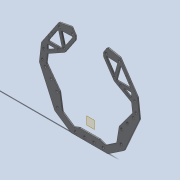
# Autodesk Inventor part: HeadMount2
Saved by Autodesk Inventor 2020 (Build 240168000, 168)
## iProperties
Created: 2021-07-03
Part Number: HeadMount2
Material: Generic
Document SubType Name: Sheet Metal
Designer: Val
Density: 1 g/cm^3
Sheet Metal Rule: Default
Appearance: Default
Author: Val
Autodesk Inventor part; units mm, degrees
ref_plane "YZ Plane" through (0, 0, 0) normal (1, 0, 0) x (0, 1, 0)
ref_plane "XZ Plane" through (0, 0, 0) normal (0, 1, 0) x (-1, 0, 0)
ref_plane "XY Plane" through (0, 0, 0) normal (0, 0, 1) x (1, 0, 0)
ref_plane "HeadMountPlane" through (0, 0, 3.048) normal (0, 0, 1) x (1, 0, 0)
sketch "Base" plane through (0, 0, 3.048) normal (0, 0, 1) x (1, 0, 0)
  line L0 (-84.8386, 199.7574) -> (-34.2356, 209.5937)
  line L1 (-34.2356, 209.5937) -> (-30.7591, 191.7089)
  line L2 (-30.7591, 191.7089) -> (-68.2682, 136.0994)
  line L3 (-68.2682, 136.0994) -> (-116.7076, 108.9972)
  line L4 (-116.7076, 108.9972) -> (-119.5296, 84.4705)
  line L5 (-119.5296, 84.4705) -> (-82.4198, 34.2032)
  line L6 (-82.4198, 34.2032) -> (-75.2404, -10.1332)
  line L7 (-44.3373, -30.9776) -> (-75.2404, -10.1332)
  line L8 (-138.9788, 78.2294) -> (-96.4615, -17.266)
  line L9 (-96.4615, -17.266) -> (-51.1674, -47.8172)
  line L10 (-44.3373, -30.9776) -> (-27.7964, -24.9572)
  line L11 (-27.7964, -24.9572) -> (0, -24.9572)
  line L12 (-51.1674, -47.8172) -> (0, -47.8172)
  line L13 (-133.255, 127.9772) -> (-138.9788, 78.2294)
  line L14 (0, -99.2994) -> (0, 261.0758) construction
  line L15 (-194.5703, 0) -> (194.5703, 0) construction
  line L16 (-84.8386, 199.7574) -> (-133.255, 127.9772)
  line L17 (84.8386, 199.7574) -> (34.2356, 209.5937)
  line L18 (34.2356, 209.5937) -> (30.7591, 191.7089)
  line L19 (30.7591, 191.7089) -> (68.2682, 136.0994)
  line L20 (68.2682, 136.0994) -> (116.7076, 108.9972)
  line L21 (116.7076, 108.9972) -> (119.5296, 84.4705)
  line L22 (119.5296, 84.4705) -> (82.4198, 34.2032)
  line L23 (82.4198, 34.2032) -> (75.2404, -10.1332)
  line L24 (44.3373, -30.9776) -> (75.2404, -10.1332)
  line L25 (138.9788, 78.2294) -> (96.4615, -17.266)
  line L26 (96.4615, -17.266) -> (51.1674, -47.8172)
  line L27 (44.3373, -30.9776) -> (27.7964, -24.9572)
  line L28 (27.7964, -24.9572) -> (0, -24.9572)
  line L29 (51.1674, -47.8172) -> (0, -47.8172)
  line L30 (133.255, 127.9772) -> (138.9788, 78.2294)
  line L31 (84.8386, 199.7574) -> (133.255, 127.9772)
  dimension "d61" = 160
  dimension "d63" = 126
  dimension "d65" = 17.78
  dimension "d66" = 22.86
  dimension "d67" = 137
  dimension "d68" = 125.791
  dimension "d70" = 34
  dimension "d71" = 11
  dimension "d74" = 83.437
  dimension "d75" = 99.198
  dimension "d76" = 114
  dimension "d77" = 24.9572
  dimension "d78" = 18.6084
  dimension "d79" = 49.3346
  dimension "d80" = 46.2853
  dimension "d81" = 82.6042
  dimension "d82" = 57.1022
  dimension "d83" = 20.7312
  dimension "d84" = 110.5412
  dimension "d85" = 116.1758
  dimension "d86" = 40.5476
  dimension "d87" = 175.1495
  dimension "d88" = 80.4922
  dimension "d89" = 197.3813
  dimension "d90" = 0
  dimension "d91" = 0
  measures "d61" angle of L11 L10
  measures "d63" angle of L10 L7
  measures "d65" distance between parallel lines of L9 L7
  measures "d66" distance between parallel lines of L12 L11
  measures "d67" angle of L4 L5
  measures "d68" angle of L3 L4
  measures "d70" angle of L14 L2
  measures "d71" angle of L14 L1
  measures "d74" angle of L15 L30
  measures "d75" angle of L15 L6
  measures "d76" angle of L15 L8
  measures "d77" distance between parallel lines of L15 L11
  measures "d78" distance between parallel lines of L21 L30
  measures "d79" distance between parallel lines of L19 L31
  measures "d80" distance from line of L15.end L30
  measures "d81" distance from line of L15.end L25
  measures "d82" distance from line of L15.end L20
  measures "d83" distance from line of L15.end L31
  measures "d84" distance from line of L15.end L22
  measures "d85" distance from line of L15.end L23
  measures "d86" distance from line of L15.end L26
  measures "d87" distance from line of L15.end L17
  measures "d88" distance from line of L15.end L27
  measures "d89" distance from line of L15.end L18
  measures "d90" distance from line of L11.end L14
  measures "d91" distance from line of L12.end L14
extrude "Plate2" add sketch "Base" along normal blind 3.175
sketch "MountHoles" plane through (0, 0, 6.223) normal (0, 0, 1) x (1, 0, 0)
  circle A0 centre (82.6068, 190.1381) radius 2.7051 construction
  circle A1 centre (126.1495, 116.4039) radius 2.7051 construction
  circle A2 centre (-126.1493, 116.4039) radius 2.7051 construction
  circle A3 centre (-82.6065, 190.1381) radius 2.2682 construction
  circle A4 centre (-82.6065, 190.1381) radius 3.175
  circle A5 centre (-126.1493, 116.4039) radius 3.175
  circle A6 centre (82.6068, 190.1381) radius 3.175
  circle A7 centre (126.1495, 116.4039) radius 3.175
  point P0 (0, 0)
  dimension "d172" = 6.35
  dimension "d173" = 6.35
  dimension "d174" = 6.35
  dimension "d175" = 6.35
  constraints: 4 centre point, 4 coincident
  measures "d172" diameter of A4
  measures "d173" diameter of A5
  measures "d174" diameter of A6
  measures "d175" diameter of A7
extrude "MountHolesFeature" cut sketch "MountHoles" against normal blind 3.175
sketch "EndCut" plane through (0, 0, 6.223) normal (0, 0, 1) x (1, 0, 0)
  line L0 (-84.8386, 199.7574) -> (-34.2356, 209.5937) projected
  line L1 (-49.4756, 206.6313) -> (-35.3576, 184.8914)
  line L2 (-30.7591, 191.7089) -> (-68.2682, 136.0994) projected
  line L3 (-34.2356, 209.5937) -> (-30.7591, 191.7089) projected
  point P0 (0, 0)
  dimension "d94" = 22
  dimension "d95" = 15.24
  constraints: 2 end point, 2 point on line
  measures "d94" angle of L3 L1
  measures "d95" horizontal distance of L0.end L1.start
extrude "EndCutFeature" cut sketch "EndCut" against normal blind 3.175
mirror "EndCutMirrorFeature" about plane through (0, 0, 0) normal (1, 0, 0) of "EndCutFeature"
sketch "Pattern" plane through (0, 0, 6.223) normal (0, 0, 1) x (1, 0, 0)
  line L0 (-27.7964, -24.9572) -> (27.7964, -24.9572) construction
  line L1 (0, -24.9572) -> (0, -47.8172)
  line L2 (51.1674, -47.8172) -> (-51.1674, -47.8172) construction
  circle A0 centre (-38.1, -39.3974) radius 3.175
  circle A1 centre (-88.1853, -6.0444) radius 3.175
  circle A2 centre (-122.5543, 75.0981) radius 3.175
  line L3 (-115.1093, 140.5729) -> (-74.9005, 140.5729)
  line L4 (-74.9005, 140.5729) -> (-86.3732, 183.1759)
  line L5 (-86.3732, 183.1759) -> (-115.1093, 140.5729)
  line L6 (-68.9795, 149.3513) -> (-78.184, 183.5316)
  line L7 (-78.184, 183.5316) -> (-44.9508, 184.9752)
  line L8 (-44.9508, 184.9752) -> (-68.9795, 149.3513)
  line L9 (-90.9552, 132.5729) -> (-116.7076, 132.5729)
  line L10 (-116.7076, 132.5729) -> (-116.7076, 118.1643)
  line L11 (-116.7076, 118.1643) -> (-90.9552, 132.5729)
  line L12 (-68.2682, 136.0994) -> (-116.7076, 108.9972) projected
  circle A3 centre (-90.0071, 31.0111) radius 3.175
  circle A4 centre (-106.2807, 53.0546) radius 3.175
  circle A5 centre (-12.7, -39.3974) radius 3.175
  line L13 (-44.3373, -30.9776) -> (-51.1674, -47.8172) construction
  line L14 (-38.1, -39.3974) -> (-12.7, -39.3974) construction
  line L15 (-51.1674, -47.8172) -> (-96.4615, -17.266) construction
  line L16 (-75.2404, -10.1332) -> (-96.4615, -17.266) construction
  line L17 (-82.4198, 34.2032) -> (-75.2404, -10.1332) construction
  line L18 (-96.4615, -17.266) -> (-138.9788, 78.2294) construction
  line L19 (-122.5543, 75.0981) -> (-90.0071, 31.0111) construction
  line L20 (-119.5296, 84.4705) -> (-82.4198, 34.2032) construction
  line L21 (-116.7076, 108.9972) -> (-119.5296, 84.4705) projected
  line L22 (-119.5296, 84.4705) -> (-138.9788, 78.2294) construction
  line L23 (-35.3576, 184.8914) -> (-68.2682, 136.0994) projected
  line L24 (-35.3576, 184.8914) -> (-49.4756, 206.6313) projected
  line L25 (-116.7076, 118.1643) -> (-116.7076, 108.9972) construction
  line L26 (-133.255, 127.9772) -> (-84.8386, 199.7574) projected
  line L27 (-84.8386, 199.7574) -> (-49.4756, 206.6313) projected
  line L28 (-74.9005, 140.5729) -> (-68.2682, 136.0994) construction
  line L29 (-86.3732, 183.1759) -> (-78.184, 183.5316) construction
  circle A6 centre (-129.2811, 89.1837) radius 3.175
  line L30 (-126.1493, 116.4039) -> (-129.2811, 89.1837) construction
  circle A7 centre (-126.1493, 116.4039) radius 3.175 projected
  circle A8 centre (-82.6065, 190.1381) radius 2.2682 projected
  point P0 (0, 0)
  dimension "d121" = 8.4198
  dimension "d122" = 8.4198
  dimension "d123" = 25.4
  dimension "d124" = 12.7
  dimension "d125" = 12.1249
  dimension "d126" = 12.1249
  dimension "d127" = 8
  dimension "d128" = 8
  dimension "d129" = 8
  dimension "d130" = 8
  dimension "d134" = 8
  dimension "d135" = 8
  dimension "d136" = 8
  dimension "d137" = 8
  dimension "d139" = 8
  dimension "d141" = 8
  dimension "d143" = 8
  dimension "d161" = 27.3997
  dimension "d162" = 27.3997
  dimension "d176" = 6.35
  dimension "d178" = 2.487
  constraints: 38 end point, 8 parallel, 7 centre point, 6 equal radius, 3 midpoint, 2 horizontal, 2 perpendicular, 1 coincident, 1 collinear, 1 vertical
  measures "d121" distance between parallel lines of L2 L14
  measures "d122" distance from line of L13.start L14
  measures "d123" distance of L14.start L14.end
  measures "d124" distance from line of L1 L14.end
  measures "d125" distance from line of L17 A1.centre
  measures "d126" distance from line of L18 A1.centre
  measures "d127" distance from line of L16 A1.centre
  measures "d128" distance from line of L17 L19.end
  measures "d129" distance between parallel lines of L20 L19
  measures "d130" distance from line of L22 L19.start
  measures "d134" distance between parallel lines of L12 L11
  measures "d135" distance between parallel lines of L3 L9
  measures "d136" distance between parallel lines of L23 L8
  measures "d137" distance between parallel lines of L4 L6
  measures "d139" distance between parallel lines of L26 L5
  measures "d141" distance from line of L24 L7.end
  measures "d143" distance of L3.end L12.start
  measures "d161" distance of A4.centre L19.start
  measures "d162" distance of L30.start L30.end
  measures "d176" diameter of A6
  measures "d178" angle of L0 L29
extrude "PatternCutFeature" cut sketch "Pattern" against normal blind 3.175 contours A0 | A1 | A2 | L5 L4 L3 | L6 L7 L8 | L11 L10 L9 | A3 | A4 | A5 | A6
mirror "PatternCutMirrorFeature" about plane through (0, 0, 0) normal (1, 0, 0) of "PatternCutFeature"
chamfer "CutChamferFeature" distance 6.35 angle 45 2 edges at (-35.3576, 184.8914, 4.6355) (35.3576, 184.8914, 4.6355)
fillet "PatternInsideFilletsFeature" radius 2 9 edges at (-68.9795, 149.3513, 4.6355) (-44.9508, 184.9752, 4.6355) (-78.184, 183.5316, 4.6355) (-116.7076, 118.1643, 4.6355) (-90.9552, 132.5729, 4.6355) (-116.7076, 132.5729, 4.6355) (-86.3732, 183.1759, 4.6355) (-115.1093, 140.5729, 4.6355) (-74.9005, 140.5729, 4.6355)
mirror "PatternInsideFilletsMirrorFeature" about plane through (0, 0, 0) normal (1, 0, 0) of "PatternInsideFilletsFeature"
fillet "BaseFilletsFeature" radius 4 15 edges at (-49.4756, 206.6313, 4.6355) (-84.8386, 199.7574, 4.6355) (-38.816, 190.217, 4.6355) (-38.9084, 179.6271, 4.6355) (-133.255, 127.9772, 4.6355) (-68.2682, 136.0994, 4.6355) (-116.7076, 108.9972, 4.6355) (-119.5296, 84.4705, 4.6355) (-138.9788, 78.2294, 4.6355) (-96.4615, -17.266, 4.6355) (-51.1674, -47.8172, 4.6355) (-82.4198, 34.2032, 4.6355) (-75.2404, -10.1332, 4.6355) (-44.3373, -30.9776, 4.6355) (-27.7964, -24.9572, 4.6355)
mirror "BaseFilletsMirrorFeature" about plane through (0, 0, 0) normal (1, 0, 0) of "BaseFilletsFeature"
sketch "ExtraMountHole" plane through (0, 0, 6.223) normal (0, 0, 1) x (1, 0, 0)
  circle A0 centre (-86.3366, 133.7771) radius 2.5
  line L0 (-39.5816, 178.629) -> (-67.7359, 136.8886) projected
  arc A1 (-70.1187, 153.5819) -> (-66.5295, 152.9835) centre (-68.1875, 154.1019) ccw projected
  arc A2 (-77.5103, 140.5729) -> (-75.5791, 143.093) centre (-77.5103, 142.5729) ccw projected
  line L1 (-70.1187, 153.5819) -> (-77.5351, 181.1217) projected
  line L2 (-85.234, 178.9453) -> (-75.5791, 143.093) projected
  line L3 (-69.0989, 135.6346) -> (-114.9209, 109.9969) projected
  line L4 (-77.5103, 140.5729) -> (-111.3478, 140.5729) projected
  arc A3 (-97.6492, 128.8276) -> (-98.6258, 132.5729) centre (-98.6258, 130.5729) ccw projected
  circle A4 centre (-69.6752, 146.1663) radius 2.5
  point P0 (0, 0)
  dimension "d151" = 6.7958
  dimension "d152" = 6.7958
  dimension "d153" = 12.7
  dimension "d160" = 5
  dimension "d179" = 6.7958
  dimension "d180" = 6.5
  constraints: 2 centre point, 1 equal radius
  measures "d151" distance from line of L3 A0.centre
  measures "d152" distance from line of L4 A0.centre
  measures "d153" distance of A3.centre A0.centre
  measures "d160" diameter of A0
  measures "d179" distance from line of L0 A4.centre
  measures "d180" distance from line of L2 A4.centre
extrude "ExtraMountHoleFeature" cut sketch "ExtraMountHole" against normal blind 3.175
mirror "ExtraMountHoleMirrorFeature" about plane through (0, 0, 0) normal (1, 0, 0) of "ExtraMountHoleFeature"
sketch "EdgeMountHole" plane through (0, 0, 6.223) normal (0, 0, 1) x (1, 0, 0)
  circle A0 centre (-46.4246, 190.9168) radius 3.175
  line L0 (-39.4717, 191.2266) -> (-48.0061, 204.3685) projected
  line L1 (-75.6906, 183.6399) -> (-48.9139, 184.803) projected
  point P0 (0, 0)
  dimension "d170" = 6
  dimension "d171" = 6
  dimension "d177" = 6.35
  constraints: 1 centre point
  measures "d170" distance from line of L0 A0.centre
  measures "d171" distance from line of L1 A0.centre
  measures "d177" diameter of A0
hole "EdgeMountHoleFeature" at (-46.4246, 190.9168, 6.223) direction (0, 0, -1) diameter 6.35 depth 3.175 tip angle 118
mirror "EdgeMountHoleMirrorFeature" about plane through (0, 0, 0) normal (1, 0, 0) of "EdgeMountHoleFeature"
sketch "BackEyeMountHoles" plane through (0, 0, 6.223) normal (0, 0, 1) x (1, 0, 0)
  circle A0 centre (102.9034, 165.822) radius 1.25 projected
  circle A1 centre (102.9034, 165.822) radius 1.25 projected
  circle A2 centre (111.8819, 152.5786) radius 1.25 projected
  point P0 (0, 0)
hole "BackEyeMountHolesFeature" at (102.9034, 165.822, 6.223) at (111.8819, 152.5786, 6.223) direction (0, 0, -1) diameter 3 end through all
mirror "BackEyeMountHolesMirrorFeature" about plane through (0, 0, 0) normal (1, 0, 0) of "BackEyeMountHolesFeature"
equation "\"d39\" = Thickness"
equation "\"BendRadius\" = Thickness"
equation "\"BendReliefWidth\" = Thickness"
equation "\"BendReliefDepth\" = 0.5 * Thickness"
equation "\"CornerReliefSize\" = 4 * Thickness"
equation "\"MinimumRemnant\" = 2 * Thickness"
equation "\"TransitionRadius\" = BendRadius"
equation "\"JacobiRadiusSize\" = BendRadius"
equation "\"GapSize\" = Thickness"
equation "\"Thickness\" = 3.175"
body "Solid1"
